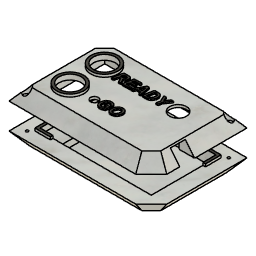
stopwatch_transmitter (Autodesk Fusion 360 design; units mm, degrees)
Autodesk Fusion 360 part; units mm, degrees
note: some values were not read from the file. Chosen so that the rebuilt part matches the saved one: which face or edge a step refers to; which sketch regions a step uses; which pieces of a blend or face edit are solid.
sketch "Sketch1" plane through (0, 0, 0) normal (0, 0, 1) x (1, 0, 0)
  line L0 (0, 0) -> (70, 0)
  line L1 (70, 0) -> (70, 50)
  line L2 (70, 50) -> (0, 50)
  line L3 (0, 50) -> (0, 0)
  line L4 (-2, -2) -> (72, -2)
  line L5 (72, -2) -> (72, 52)
  line L6 (72, 52) -> (-2, 52)
  line L7 (-2, 52) -> (-2, -2)
  line L8 (0, 50) -> (-14, 50)
  line L9 (-14, 50) -> (-14, 0)
  line L10 (-14, 0) -> (0, 0)
  line L11 (0, 0) -> (0, 50)
  line L12 (2, 52) -> (-16, 52)
  line L13 (-16, 52) -> (-16, -2)
  line L14 (-16, -2) -> (2, -2)
  dimension "d1" = 70
  dimension "d2" = 50
  dimension "d3" = 2
  dimension "d10" = 14
  constraint horizontal L0
  constraint vertical L1
  constraint horizontal L2
  constraint vertical L3
  constraint coincident L0.start L3.end
  constraint horizontal L8
  constraint vertical L9
  constraint horizontal L10
  constraint vertical L11
  measures "d1" distance of L0.start L0.end
  measures "d2" distance of L0.start L2.end
  measures "d10" distance of L2.end L8.end
extrude "Extrude1" add sketch "Sketch1" along normal blind 2 contours L0 L1 L2 L3 L11 makes body 1
extrude "Extrude2" add sketch "Sketch1" along normal blind 5 contours L3 L7 L8 L10 L11 | L0 L1 L2 L4 L5 L6 L7 L8 L10 L12 L14 bodies 1
extrude "Extrude3" add 1 faces at (46.6667, -1.3333, 5) along direction (0, 0, 1) blind 2 on bodies 1 bodies 1
extrude "Extrude4" add sketch "Sketch1" along normal blind 8 contours L7 L8 L9 L10 L12 L13 L14 bodies 1
extrude "Extrude5" add sketch "Sketch1" along normal blind 7 contours L7 L8 L9 L10 bodies 1
sketch "Sketch2" plane through (0, 0, 7) normal (0, 0, 1) x (-1, 0, 0)
  line L0 (0, 0) -> (0, -50)
  line L1 (0, -50) -> (-70, -50)
  line L2 (-70, -50) -> (-70, 0)
  line L3 (-70, 0) -> (0, 0)
  line L4 (2, -52) -> (2, -50)
  line L5 (2, -50) -> (14, -50)
  line L6 (14, -50) -> (14, 0)
  line L7 (14, 0) -> (2, 0)
  line L8 (2, 0) -> (2, 2)
  line L9 (2, 2) -> (-72, 2)
  line L10 (-72, 2) -> (-72, -52)
  line L11 (-72, -52) -> (2, -52)
  line L12 (0, 0) -> (2, 0)
  line L13 (0, -50) -> (2, -50)
  constraint coincident L0.start L3.end
  constraint coincident L7.end L8.start
  constraint coincident L0.end L1.start
  constraint coincident L4.end L5.start
extrude "Extrude6" add sketch "Sketch2" along normal blind 1 contours L1 L2 L3 L4 L8 L9 L10 L11 L12 L13 bodies 1
extrude "Extrude7" add 1 faces at (72, 16, 2.6667) along direction (1, 0, 0) blind 1 on bodies 1 bodies 1
sketch "Sketch3" plane through (0, 0, 8) normal (0, 0, 1) x (-1, 0, 0)
  line L0 (-73, -52) -> (16, -52)
  line L1 (16, -52) -> (16, 2)
  line L2 (16, 2) -> (-73, 2)
  line L3 (-73, 2) -> (-73, -52)
  line L4 (14, -50) -> (-70, -50)
  line L5 (-70, -50) -> (-70, 0)
  line L6 (-70, 0) -> (14, 0)
  line L7 (14, 0) -> (14, -50)
  line L8 (-70, -50) -> (-71, -50)
  line L9 (-71, -50) -> (-71, 0)
  line L10 (-71, 0) -> (-70, 0)
  line L11 (-70, 0) -> (-70, -50)
  line L12 (-70, -50) -> (-71, -50)
  line L13 (-71, -50) -> (-71, -30)
  line L14 (-71, -30) -> (-70, -30)
  line L15 (-70, -30) -> (-70, -50)
  line L16 (-71, 0) -> (-70, 0)
  line L17 (-70, 0) -> (-70, -20)
  line L18 (-70, -20) -> (-71, -20)
  line L19 (-71, -20) -> (-71, 0)
  dimension "d20" = 1
  dimension "d21" = 20
  constraint horizontal L8
  constraint vertical L9
  constraint horizontal L10
  constraint vertical L11
  constraint coincident L4.end L5.start
  constraint horizontal L12
  constraint vertical L13
  constraint horizontal L14
  constraint vertical L15
  constraint coincident L9 L13.end
  constraint horizontal L16
  constraint vertical L17
  constraint horizontal L18
  constraint vertical L19
  measures "d20" distance of L4.end L8.end
  measures "d21" distance of L9.end L18.end
extrude "Extrude8" cut sketch "Sketch3" against normal blind 1 contours L5 L8 L9 L11 L12 L13 L14 L15 | L5 L9 L10 L11 L16 L17 L18 L19 bodies 1
extrude "Extrude9" cut sketch "Sketch3" against normal blind 6 contours L5 L9 L11 L14 L18 bodies 1
extrude "Extrude10" add 1 faces at (73, 16, 2.6667) along direction (1, 0, 0) blind 1 on bodies 1 bodies 1
extrude "Extrude11" cut 1 faces at (71, 26.6667, 3.6667) along direction (1, 0, 0) blind 1 on bodies 1 bodies 1
sketch "Sketch4" plane through (0, 0, 8) normal (0, 0, 1) x (-1, 0, 0)
  line L0 (-72, 0) -> (14, 0)
  line L1 (14, 0) -> (14, -50)
  line L2 (14, -50) -> (-72, -50)
  line L3 (-72, -50) -> (-72, 0)
  line L4 (-74, -52) -> (16, -52)
  line L5 (16, -52) -> (16, 2)
  line L6 (16, 2) -> (-74, 2)
  line L7 (-74, 2) -> (-74, -52)
  line L8 (16, -52) -> (-74, -52)
  line L9 (-74, 2) -> (16, 2)
  line L10 (16, 2) -> (16, -52)
  line L11 (-74, 2) -> (-74, 1.5)
  line L12 (-74, 2) -> (-74, -10)
  line L13 (-74, -52) -> (-74, -21)
  line L14 (-74, -21) -> (-72, -21)
  line L15 (-72, -21) -> (-72, -10)
  line L16 (-72, -10) -> (-74, -10)
  line L17 (16, -52) -> (-10.5, -52)
  line L18 (-74, -52) -> (-19.5, -52)
  line L19 (-10.5, -52) -> (-19.5, -52)
  line L20 (-19.5, -52) -> (-19.5, -50)
  line L21 (-19.5, -50) -> (-10.5, -50)
  line L22 (-10.5, -50) -> (-10.5, -52)
  line L23 (16, -52) -> (16, -47)
  line L24 (16, 2) -> (16, -3)
  line L25 (16, -25) -> (16, -30)
  line L26 (16, -25) -> (16, -20)
  line L27 (16, 2) -> (15, 2)
  line L28 (16, 2) -> (11, 2)
  line L29 (16, -52) -> (11, -52)
  line L30 (-74, -52) -> (-73.5, -52)
  line L31 (-74, -52) -> (-63, -52)
  line L32 (-74, -52) -> (-74, -42)
  line L33 (16, 2) -> (-12, 2)
  line L34 (16, 2) -> (16, -9)
  line L35 (2.5, -38.5) -> (2.5, -38.25)
  circle A0 centre (2.5, -38.25) radius 8.5
  line L36 (2.5, -11.5) -> (2.5, -11.75)
  circle A1 centre (2.5, -11.75) radius 8.5
  line L37 (-15, -12) -> (-16, -12)
  line L38 (-56.5, -35.5) -> (-56.5, -36.5)
  line L39 (-56.5, -36.5) -> (-56.25, -36.5)
  circle A2 centre (-56.25, -36.5) radius 6.5
  circle A3 centre (-16, -12) radius 3
  line L40 (-8.9387, -32.2692) -> (-47.6004, -32.6117) construction
  line L41 (-47.6004, -32.6117) -> (-47.5301, -40.5565) construction
  line L42 (-47.5301, -40.5565) -> (-8.8683, -40.214) construction
  line L43 (-8.8683, -40.214) -> (-8.9387, -32.2692) construction
  line L44 (-20.8588, -8.0842) -> (-38.0381, -8.2489) construction
  line L45 (-38.0381, -8.2489) -> (-37.9619, -16.1956) construction
  line L46 (-37.9619, -16.1956) -> (-20.7826, -16.0308) construction
  line L47 (-20.7826, -16.0308) -> (-20.8588, -8.0842) construction
  circle A4 centre (2.5, -38.25) radius 10.5
  circle A5 centre (2.5, -11.75) radius 10.5
  dimension "d30" = 12
  dimension "d31" = 31
  dimension "d32" = 26.5
  dimension "d33" = 54.5
  dimension "d34" = 5
  dimension "d35" = 5
  dimension "d36" = 5
  dimension "d37" = 5
  dimension "d38" = 5
  dimension "d41" = 5
  dimension "d44" = 11
  dimension "d45" = 10
  dimension "d48" = 28
  dimension "d49" = 11
  dimension "d58" = 0.25
  dimension "d59" = 17
  dimension "d60" = 0.25
  dimension "d61" = 17
  dimension "d64" = 1
  dimension "d65" = 1
  dimension "d66" = 0.25
  dimension "d67" = 13
  dimension "d68" = 6
  dimension "d75" = 8
  dimension "d76" = 8
  dimension "d77" = 2
  dimension "d78" = 2
  text T0 "READY" font "Arial" height 8 bold italic align left top in box 38.6633 x 7.9451 at (-8.9387, -32.2692) x (-0.999961, -0.00886) y (0.00886, -0.999961) spacing 1
  text T1 "GO" font "Arial" height 8 bold italic align left top in box 17.1801 x 7.947 at (-20.8588, -8.0842) x (-0.999954, -0.00959) y (0.00959, -0.999954) spacing 1
  constraint horizontal L8
  constraint horizontal L9
  constraint vertical L10
  constraint coincident L6.end L7.start
  constraint coincident L4.end L5.start
  constraint perpendicular L9 L12
  constraint perpendicular L4 L13
  constraint horizontal L14
  constraint vertical L15
  constraint horizontal L16
  constraint coincident L3 L15.end
  constraint perpendicular L1 L17
  constraint perpendicular L13 L18
  constraint horizontal L19
  constraint vertical L20
  constraint horizontal L21
  constraint vertical L22
  constraint coincident L2 L20.end
  constraint perpendicular L17 L23
  constraint coincident L5.end L6.start
  constraint perpendicular L0 L24
  constraint midpoint L10 L25.start
  constraint parallel L10 L25
  constraint parallel L5 L26
  constraint coincident L9 L27.end
  constraint perpendicular L10 L27
  constraint perpendicular L10 L28
  constraint perpendicular L10 L29
  constraint coincident L18 L30.end
  constraint perpendicular L13 L30
  constraint coincident L4.start L7.end
  constraint perpendicular L7 L31
  constraint perpendicular L31 L32
  constraint perpendicular L24 L33
  constraint perpendicular L0 L34
  constraint vertical L35
  constraint coincident L35.end A0.centre
  constraint vertical L36
  constraint coincident L36.end A1.centre
  constraint horizontal L37
  constraint vertical L38
  constraint perpendicular L38 L39
  constraint coincident L39.end A2.centre
  constraint coincident L37.end A3.centre
  measures "d30" distance of L6.end L12.end
  measures "d31" distance of L4.start L13.end
  measures "d32" distance of L4.end L17.end
  measures "d33" distance of L4.start L18.end
  measures "d34" distance of L4.end L23.end
  measures "d35" distance of L5.end L24.end
  measures "d36" distance of L25.start L25.end
  measures "d37" distance of L25.start L26.end
  measures "d38" distance of L5.end L28.end
  measures "d41" distance of L4.end L29.end
  measures "d44" distance of L4.start L31.end
  measures "d45" distance of L4.start L32.end
  measures "d48" distance of L5.end L33.end
  measures "d49" distance of L5.end L34.end
  measures "d58" distance of L35.start L35.end
  measures "d59" diameter of A0
  measures "d60" distance of L36.start L36.end
  measures "d61" diameter of A1
  measures "d64" distance of L37.start L37.end
  measures "d65" distance of L38.start L38.end
  measures "d66" distance of L38.end L39.end
  measures "d67" diameter of A2
  measures "d68" diameter of A3
extrude "Extrude12" add sketch "Sketch4" along normal blind 2 separate body contours L0 L1 L2 L3 L4 L5 L6 L7 L8 L9 L10 L11 L12 L16 L17 L22 L23 L24 L25 L26 L27 L28 L29 L33 L34 | L0 L1 L2 L3 L15 L21 | L2 L3 L4 L7 L8 L13 L14 L18 L20 L30 L31 L32 | A0 | A1 | A2 | A3 | A4 | A5 makes body 2
extrude "Extrude13" cut 1 faces at (73.3333, 21, 8.6667) along direction (0, 1, 0) blind 0.5 on bodies 2 bodies 2
extrude "Extrude14" add sketch "Sketch4" along normal blind 2 contours A5 bodies 2
extrude "Extrude15" add sketch "Sketch4" along normal blind 2 contours A5 bodies 2
extrude "Extrude16" cut sketch "Sketch4" along normal blind 16 contours A0 | A1 | A2 | A3 bodies 2
extrude "Extrude17" add 1 faces at (0, 33.3333, 3.6667) along direction (1, 0, 0) blind 1 on bodies 1 bodies 1
extrude "Extrude18" add 1 faces at (14.6667, -1.3333, 8) along direction (0, 0, 1) blind 0.5 on bodies 1 bodies 1
extrude "Extrude19" add sketch "Sketch4" sketch "Sketch4" along normal blind 3 contours A4 | A5 of sketch 2 text T0 T1 bodies 2
extrude "Extrude20" add 2 faces at (-12.2942, 38.7716, 11) (-12.2626, 12.6939, 11) along direction (0, 0, 1) blind 1 on bodies 2 bodies 2
move_body "Move1" bodies 2 to x (1, 0, 0) y (0, 1, 0) z (0, 0, 1) at (0, 0, 9)
extrude "Extrude21" add sketch "Sketch4" along normal blind 9 separate body contours L0 L1 L2 L3 L4 L5 L6 L7 L8 L9 L10 L11 L12 L16 L17 L22 L23 L24 L25 L26 L27 L28 L29 L33 L34 | L2 L3 L4 L7 L8 L13 L14 L18 L20 L30 L31 L32 makes body 3 at (14, -2, 14) makes body 4 at (55.8333, 52, 11)
combine "Combine1" operation add target body 3 tool bodies 2 4
extrude "Extrude22" cut 1 faces at (73.3333, 21, 11) along direction (0, 1, 0) blind 0.5 on bodies 3 bodies 3
extrude "Extrude23" add 2 faces at (72, 17.3333, 18.3333) (72, 21.1667, 17.6667) along direction (1, 0, 0) blind 2 on bodies 3 bodies 3
extrude "Extrude24" add 1 faces at (13.5, 50, 17.6667) along direction (0, 1, 0) blind 2 on bodies 3 bodies 3
move_body "Move2" bodies 3 to x (1, 0, 0) y (0, 1, 0) z (0, 0, 1) at (0, 0, 5)
extrude "Extrude25" add 1 faces at (14.6667, -1.3333, 8.5) along direction (0, 0, 1) blind 1 on bodies 1 bodies 1
move_body "Move3" bodies 1 to x (1, 0, 0) y (0, 1, 0) z (0, 0, 1) at (0, 0, -3)
extrude "Extrude26" cut sketch "Sketch4" against normal blind 2.5 contours L3 L7 L14 L15 L16 bodies 1
extrude "Extrude27" cut 1 faces at (73.3333, 21, 6.1667) along direction (0, 1, 0) blind 0.5 on bodies 1 bodies 1
extrude "Extrude28" cut 2 faces at (43.3333, -1.3333, 13) (55.1667, 51.3333, 13) along direction (0, 0, 1) blind 1 on bodies 3 bodies 3
extrude "Extrude29" add 1 faces at (44, 16, -3) along direction (0, 0, -1) blind 0.5 on bodies 1 bodies 1
extrude "Extrude30" cut sketch "Sketch4" against normal blind 3 contours L2 L4 L8 L19 L20 L21 L22 bodies 1
sketch "Sketch5" plane through (0, 0, 22) normal (0, 0, -1) x (1, 0, 0)
  circle A0 centre (56.25, -36.5) radius 6.5
  circle A1 centre (16, -12) radius 3
  circle A2 centre (-2.5, -11.75) radius 8.5
  circle A3 centre (-2.5, -38.25) radius 8.5
  line L0 (19.5, -50) -> (72, -50)
  line L1 (72, -50) -> (72, -21.5)
  line L2 (72, -21.5) -> (74, -21.5)
  line L3 (74, -21.5) -> (74, -10)
  line L4 (74, -10) -> (72, -10)
  line L5 (72, -10) -> (72, 0)
  line L6 (72, 0) -> (-14, 0)
  line L7 (-14, 0) -> (-14, -50)
  line L8 (-14, -50) -> (10.5, -50)
  line L9 (10.5, -50) -> (10.5, -52)
  line L10 (10.5, -52) -> (19.5, -52)
  line L11 (19.5, -52) -> (19.5, -50)
  line L12 (19.5, -52) -> (10.5, -52)
  line L13 (10.5, -52) -> (10.5, -50)
  line L14 (10.5, -50) -> (19.5, -50)
  line L15 (19.5, -50) -> (19.5, -52)
  constraint horizontal L12
  constraint vertical L13
  constraint horizontal L14
  constraint vertical L15
  constraint coincident L8.end L9.start
  constraint coincident L10.end L11.start
extrude "Extrude31" add sketch "Sketch5" along normal blind 0.5 contours L9 L10 L11 L12 L13 L14 L15 bodies 3
move_body "Move4" bodies 3 to x (1, 0, 0) y (0, 1, 0) z (0, 0, 1) at (0, 0, -7.5)
extrude "Extrude32" add 1 faces at (13.5, 50.6667, 14) along direction (0, 0, -1) blind 2 on bodies 3 bodies 3
extrude "Extrude33" add 1 faces at (19.5, 51.3333, 8.3333) along direction (-1, 0, 0) blind 1 on bodies 3 bodies 3
extrude "Extrude34" add 1 faces at (10.5, 50.6667, 8.3333) along direction (1, 0, 0) blind 1 on bodies 3 bodies 3
extrude "Extrude35" add 1 faces at (19.5, 51.3333, 6) along direction (-1, 0, 0) blind 1 on bodies 1 bodies 1
extrude "Extrude36" add 1 faces at (10.5, 50.6667, 6) along direction (1, 0, 0) blind 1 on bodies 1 bodies 1
extrude "Extrude37" cut 1 faces at (11.5, 50.6667, 6) along direction (-1, 0, 0) blind 0.5 on bodies 1 bodies 1
extrude "Extrude38" add 1 faces at (11, 50.6667, 6) along direction (1, 0, 0) blind 0.25 on bodies 1 bodies 1
extrude "Extrude39" cut 1 faces at (11.5, 50.6667, 8.3333) along direction (-1, 0, 0) blind 0.25 on bodies 3 bodies 3
extrude "Extrude40" add 1 faces at (73.3333, 17.5, 5.5) along direction (0, 0, 1) blind 1 on bodies 1 bodies 1
extrude "Extrude41" add 1 faces at (14, -2, 9.8333) along direction (0, -1, 0) blind 10 on bodies 3 bodies 3
extrude "Extrude42" add 4 faces at (74, -4.6667, 12.5) (74, 13.6667, 15.8333) (74, 41.8333, 12.5) (74, 21.3333, 15.8333) along direction (1, 0, 0) blind 10 on bodies 3 bodies 3
extrude "Extrude43" add 1 faces at (62.1667, 52, 11.6667) along direction (0, 1, 0) blind 10 on bodies 3 bodies 3
extrude "Extrude44" add 1 faces at (-16, 37.3333, 13.1667) along direction (-1, 0, 0) blind 10 on bodies 3 bodies 3
chamfer "Chamfer1" distance 12 angle 45 2 edges at (84, -12, 11.5) (-26, 62, 11.5) on bodies 3
chamfer "Chamfer2" distance 8 distance2 10 6 edges at (23, -12, 16.5) (78, -6, 16.5) (84, 31, 16.5) (35, 62, 16.5) (-20, 56, 16.5) (-26, 19, 16.5) measured on face at (35.4296, 54.819, 16.5) measured on face at (80, -4, 13.1667) measured on face at (35.4296, 54.819, 16.5) measured on face at (35.4296, 54.819, 16.5) measured on face at (-22, 54, 9.8333) measured on face at (-26, 8.6667, 9.8333) on bodies 3
move_face "OffsetFaces1" offset 10 4 faces at (44, -2, -0.1667) (74, 34, 3.1667) (55.5, 52, 2.6667) (-16, 34, -0.1667) on bodies 1
chamfer "Chamfer3" distance 12 distance2 12 2 edges at (-26, 62, 1.5) (84, -12, 1.5) measured on face at (62.1667, 62, 2.6667) measured on face at (10.6667, -12, 3.1667) on bodies 1
chamfer "Chamfer4" distance 8 distance2 10 6 edges at (23, -12, -3.5) (78, -6, -3.5) (84, 31, -3.5) (35, 62, -3.5) (-20, 56, -3.5) (-26, 19, -3.5) measured on face at (47.3333, 37.3333, -3.5) measured on face at (80, -4, -0.1667) measured on face at (47.3333, 37.3333, -3.5) measured on face at (47.3333, 37.3333, -3.5) measured on face at (-18, 58, -0.1667) measured on face at (47.3333, 37.3333, -3.5) on bodies 1
move_body "Move5" bodies 3 to x (1, 0, 0) y (0, 1, 0) z (0, 0, 1) at (0, 0, 20)
sketch "Sketch6" plane through (0, 0, 6.5) normal (0, 0, 1) x (-1, 0, 0)
  line L0 (-72, 12) -> (-84, 0)
  line L1 (-84, 0) -> (-84, -62)
  line L2 (-84, -62) -> (-18.5, -62)
  line L3 (-18.5, -62) -> (-18.5, -50)
  line L4 (-18.5, -50) -> (-72, -50)
  line L5 (-72, -50) -> (-72, 0)
  line L6 (-72, 0) -> (14, 0)
  line L7 (14, 0) -> (14, -50)
  line L8 (14, -50) -> (-11.25, -50)
  line L9 (-11.25, -50) -> (-11.25, -62)
  line L10 (-11.25, -62) -> (14, -62)
  line L11 (14, -62) -> (26, -50)
  line L12 (26, -50) -> (26, 12)
  line L13 (26, 12) -> (-72, 12)
  line L14 (14, 0) -> (16, 0)
  line L15 (16, 0) -> (16, -10)
  line L16 (16, -10) -> (14, -10)
  line L17 (14, -10) -> (14, 0)
  line L18 (16, 0) -> (4, 0)
  line L19 (4, 0) -> (4, 2)
  line L20 (4, 2) -> (16, 2)
  line L21 (16, 2) -> (16, 0)
  line L22 (-72, -50) -> (-62, -50)
  line L23 (-62, -50) -> (-62, -52)
  line L24 (-62, -52) -> (-72, -52)
  line L25 (-72, -52) -> (-72, -50)
  line L26 (-72, -52) -> (-74, -52)
  line L27 (-74, -52) -> (-74, -40)
  line L28 (-74, -40) -> (-72, -40)
  line L29 (-72, -40) -> (-72, -52)
  dimension "d139" = 2
  dimension "d140" = 10
  dimension "d141" = 12
  dimension "d142" = 2
  dimension "d143" = 10
  dimension "d144" = 2
  dimension "d145" = 2
  dimension "d146" = 12
  constraint horizontal L14
  constraint vertical L15
  constraint horizontal L16
  constraint vertical L17
  constraint coincident L6.end L7.start
  constraint horizontal L18
  constraint vertical L19
  constraint horizontal L20
  constraint vertical L21
  constraint horizontal L22
  constraint vertical L23
  constraint horizontal L24
  constraint vertical L25
  constraint coincident L4.end L5.start
  constraint horizontal L26
  constraint vertical L27
  constraint horizontal L28
  constraint vertical L29
  measures "d139" distance of L6.end L14.end
  measures "d140" distance of L6.end L16.end
  measures "d141" distance of L14.end L18.end
  measures "d142" distance of L14.end L20.end
  measures "d143" distance of L4.end L22.end
  measures "d144" distance of L4.end L24.end
  measures "d145" distance of L24.end L26.end
  measures "d146" distance of L24.end L28.end
extrude "Extrude45" add sketch "Sketch6" along normal blind 2 contours L7 L14 L15 L16 L17 L18 | L6 L14 L18 L19 L20 L21 bodies 1
extrude "Extrude46" add sketch "Sketch6" along normal blind 2 contours L4 L22 L23 L24 L25 L29 | L5 L25 L26 L27 L28 L29 bodies 1
extrude "Extrude47" cut sketch "Sketch6" along normal blind 28 contours L4 L22 L23 L24 L25 L29 | L5 L25 L26 L27 L28 L29 | L7 L14 L15 L16 L17 L18 | L6 L14 L18 L19 L20 L21 bodies 3
extrude "Extrude48" cut 1 faces at (-15.3333, 10, 29.1667) along direction (0, 1, 0) blind 1 on bodies 3 bodies 3
extrude "Extrude49" cut 1 faces at (-4, -0.6667, 29.1667) along direction (1, 0, 0) blind 1 on bodies 3 bodies 3
extrude "Extrude50" cut 1 faces at (62, 50.6667, 29.1667) along direction (-1, 0, 0) blind 1 on bodies 3 bodies 3
extrude "Extrude51" cut 1 faces at (73.3333, 40, 29.1667) along direction (0, -1, 0) blind 1 on bodies 3 bodies 3
sketch "Sketch7" plane through (0, 0, 6.5) normal (0, 0, 1) x (-1, 0, 0)
  line L0 (-62, -50) -> (-62, -52)
  line L1 (-62, -52) -> (-74, -52)
  line L2 (-74, -52) -> (-74, -40)
  line L3 (-74, -40) -> (-72, -40)
  line L4 (-72, -40) -> (-72, 0)
  line L5 (-72, 0) -> (4, 0)
  line L6 (4, 0) -> (4, 2)
  line L7 (4, 2) -> (16, 2)
  line L8 (16, 2) -> (16, -10)
  line L9 (16, -10) -> (14, -10)
  line L10 (14, -10) -> (14, -50)
  line L11 (14, -50) -> (-11.25, -50)
  line L12 (-11.25, -50) -> (-11.25, -62)
  line L13 (-11.25, -62) -> (14, -62)
  line L14 (14, -62) -> (26, -50)
  line L15 (26, -50) -> (26, 12)
  line L16 (26, 12) -> (-72, 12)
  line L17 (-72, 12) -> (-84, 0)
  line L18 (-84, 0) -> (-84, -62)
  line L19 (-84, -62) -> (-18.5, -62)
  line L20 (-18.5, -62) -> (-18.5, -50)
  line L21 (-18.5, -50) -> (-62, -50)
  line L22 (16, 2) -> (22, 2)
  line L23 (22, 2) -> (22, 8)
  line L24 (22, 8) -> (16, 8)
  line L25 (16, 8) -> (16, 2)
  circle A0 centre (19, 5) radius 1
  circle A1 centre (19, 5) radius 3
  line L26 (-74, -52) -> (-80, -52)
  line L27 (-80, -52) -> (-80, -58)
  line L28 (-80, -58) -> (-74, -58)
  line L29 (-74, -58) -> (-74, -52)
  circle A2 centre (-77, -55) radius 1
  circle A3 centre (-77, -55) radius 3
  dimension "d161" = 6
  dimension "d162" = 6
  dimension "d163" = 2
  dimension "d164" = 6
  dimension "d165" = 6
  dimension "d166" = 2
  constraint horizontal L22
  constraint vertical L23
  constraint horizontal L24
  constraint vertical L25
  constraint coincident L7.end L8.start
  constraint concentric A0 A1
  constraint tangent L25 A1
  constraint horizontal L26
  constraint vertical L27
  constraint horizontal L28
  constraint vertical L29
  constraint coincident L1.end L2.start
  constraint concentric A2 A3
  constraint tangent L27 A3
  measures "d161" distance of L7.end L22.end
  measures "d162" distance of L7.end L24.end
  measures "d163" diameter of A0
  measures "d164" distance of L1.end L26.end
  measures "d165" distance of L1.end L28.end
  measures "d166" diameter of A2
extrude "Extrude52" cut sketch "Sketch7" against normal blind 4 contours A0 bodies 1
extrude "Extrude53" cut sketch "Sketch7" against normal blind 4 contours A2 bodies 1
extrude "Extrude54" cut sketch "Sketch7" along normal blind 57 contours A0 | A2 bodies 3
sketch "Sketch8" plane through (0, 0, 36.5) normal (0, 0, 1) x (-1, 0, 0)
  line L0 (-10.5871, -32.2289) -> (-8.9392, -32.2143)
  line L1 (-8.9392, -32.2143) -> (-10.5435, -40.2288)
  line L2 (-10.5435, -40.2288) -> (-14.0959, -40.2603)
  spline S0 degree 3 poles (-14.0959, -40.2603) (-14.3379, -40.2599) (-14.5799, -40.2596) (-15.0631, -40.2046) (-15.2587, -40.1538) (-15.5245, -40.0847) knots 0 0 0 0 0.072595 0.072595 0.147152 0.147152 0.147152 0.147152
  spline S1 degree 3 poles (-15.5245, -40.0847) (-15.699, -40.0034) (-15.8595, -39.9287) (-16.1355, -39.6999) (-16.245, -39.5508) (-16.3546, -39.4017) knots 0 0 0 0 0.05773 0.05773 0.115402 0.115402 0.115402 0.115402
  spline S2 degree 3 poles (-16.3546, -39.4017) (-16.4602, -39.1966) (-16.5501, -39.022) (-16.6558, -38.6156) (-16.6675, -38.4016) (-16.6792, -38.1876) knots 0 0 0 0 0.069205 0.069205 0.138098 0.138098 0.138098 0.138098
  spline S3 degree 3 poles (-16.6792, -38.1876) (-16.6609, -37.8769) (-16.6425, -37.5662) (-16.4471, -37.0013) (-16.2758, -36.7649) (-16.0829, -36.4987) knots 0 0 0 0 0.093372 0.093372 0.18695 0.18695 0.18695 0.18695
  spline S4 degree 3 poles (-16.0829, -36.4987) (-15.7851, -36.2497) (-15.5518, -36.0546) (-14.9295, -35.7821) (-14.5849, -35.7216) (-14.2403, -35.6611) knots 0 0 0 0 0.116479 0.116479 0.231434 0.231434 0.231434 0.231434
  spline S5 degree 3 poles (-14.2403, -35.6611) (-14.365, -35.5388) (-14.4682, -35.4374) (-14.6683, -35.1883) (-14.755, -35.0536) (-14.8418, -34.9188) knots 0 0 0 0 0.052389 0.052389 0.104433 0.104433 0.104433 0.104433
  spline S6 degree 3 poles (-14.8418, -34.9188) (-15.1074, -34.4325) (-15.3033, -34.074) (-15.7224, -33.1803) (-15.9077, -32.729) (-16.093, -32.2777) knots 0 0 0 0 0.166241 0.166241 0.328188 0.328188 0.328188 0.328188
  line L3 (-16.093, -32.2777) -> (-14.325, -32.262)
  spline S7 degree 3 poles (-14.325, -32.262) (-14.177, -32.6697) (-14.0732, -32.9555) (-13.7789, -33.6741) (-13.6252, -34.0202) (-13.4714, -34.3664) knots 0 0 0 0 0.130111 0.130111 0.253846 0.253846 0.253846 0.253846
  spline S8 degree 3 poles (-13.4714, -34.3664) (-13.3816, -34.5624) (-13.2918, -34.7583) (-13.0498, -35.1139) (-12.921, -35.2345) (-12.7419, -35.4023) knots 0 0 0 0 0.064675 0.064675 0.131653 0.131653 0.131653 0.131653
  spline S9 degree 3 poles (-12.7419, -35.4023) (-12.5926, -35.4652) (-12.4876, -35.5095) (-12.2064, -35.5556) (-12.0642, -35.5544) (-11.922, -35.5532) knots 0 0 0 0 0.048618 0.048618 0.094938 0.094938 0.094938 0.094938
  line L4 (-11.922, -35.5532) -> (-11.2508, -35.5473)
  line L5 (-11.2508, -35.5473) -> (-10.5871, -32.2289)
  line L6 (-44.594, -32.5302) -> (-42.9515, -32.5156)
  line L7 (-42.9515, -32.5156) -> (-43.5732, -35.6372)
  line L8 (-43.5732, -35.6372) -> (-41.3254, -40.5016)
  line L9 (-41.3254, -40.5016) -> (-43.077, -40.5171)
  line L10 (-43.077, -40.5171) -> (-44.0902, -38.2668)
  spline S10 degree 3 poles (-44.0902, -38.2668) (-44.1764, -38.0741) (-44.2626, -37.8815) (-44.4301, -37.4811) (-44.4898, -37.3236) (-44.5753, -37.0977) knots 0 0 0 0 0.063314 0.063314 0.130264 0.130264 0.130264 0.130264
  spline S11 degree 3 poles (-44.5753, -37.0977) (-44.6538, -37.2346) (-44.7223, -37.354) (-44.8769, -37.6067) (-44.9574, -37.7308) (-45.0379, -37.8549) knots 0 0 0 0 0.047317 0.047317 0.094492 0.094492 0.094492 0.094492
  line L11 (-45.0379, -37.8549) -> (-45.7871, -38.9203)
  line L12 (-45.7871, -38.9203) -> (-46.9023, -40.551)
  line L13 (-46.9023, -40.551) -> (-48.8121, -40.5679)
  line L14 (-48.8121, -40.5679) -> (-45.1898, -35.4988)
  line L15 (-45.1898, -35.4988) -> (-44.594, -32.5302)
  line L16 (-29.6539, -34.166) -> (-26.4835, -34.1379)
  line L17 (-26.4835, -34.1379) -> (-25.5388, -32.3614)
  line L18 (-25.5388, -32.3614) -> (-23.8472, -32.3464)
  line L19 (-23.8472, -32.3464) -> (-28.3, -40.3861)
  line L20 (-28.3, -40.3861) -> (-30.128, -40.4023)
  line L21 (-30.128, -40.4023) -> (-31.4976, -32.4142)
  line L22 (-31.4976, -32.4142) -> (-29.937, -32.4003)
  line L23 (-29.937, -32.4003) -> (-29.6539, -34.166)
  line L24 (-16.977, -32.2855) -> (-18.5759, -40.3)
  line L25 (-18.5759, -40.3) -> (-24.5075, -40.3525)
  line L26 (-24.5075, -40.3525) -> (-24.241, -39.0131)
  line L27 (-24.241, -39.0131) -> (-19.9574, -38.9752)
  line L28 (-19.9574, -38.9752) -> (-19.5916, -37.1547)
  line L29 (-19.5916, -37.1547) -> (-23.7333, -37.1914)
  line L30 (-23.7333, -37.1914) -> (-23.4668, -35.852)
  line L31 (-23.4668, -35.852) -> (-19.3251, -35.8153)
  line L32 (-19.3251, -35.8153) -> (-18.8423, -33.639)
  line L33 (-18.8423, -33.639) -> (-23.497, -33.6803)
  line L34 (-23.497, -33.6803) -> (-23.2251, -32.3409)
  line L35 (-23.2251, -32.3409) -> (-16.977, -32.2855)
  circle A0 centre (-56.25, -36.5) radius 6.5
  circle A1 centre (-16, -12) radius 3
  spline S12 degree 3 poles (-29.5109, -11.2521) (-29.5194, -11.5197) (-29.5269, -11.7571) (-29.5942, -12.2566) (-29.6518, -12.503) (-29.7094, -12.7493) knots 0 0 0 0 0.080324 0.080324 0.160466 0.160466 0.160466 0.160466
  spline S13 degree 3 poles (-29.7094, -12.7493) (-29.8049, -13.075) (-29.9004, -13.4006) (-30.1759, -14.014) (-30.3481, -14.2839) (-30.5404, -14.5855) knots 0 0 0 0 0.101809 0.101809 0.203811 0.203811 0.203811 0.203811
  spline S14 degree 3 poles (-30.5404, -14.5855) (-30.7436, -14.8355) (-30.9435, -15.0815) (-31.4191, -15.4942) (-31.6928, -15.6593) (-31.9665, -15.8243) knots 0 0 0 0 0.096655 0.096655 0.193306 0.193306 0.193306 0.193306
  spline S15 degree 3 poles (-31.9665, -15.8243) (-32.2978, -15.9707) (-32.5936, -16.1014) (-33.2519, -16.2555) (-33.5947, -16.2744) (-33.9376, -16.2934) knots 0 0 0 0 0.10865 0.10865 0.217084 0.217084 0.217084 0.217084
  spline S16 degree 3 poles (-33.9376, -16.2934) (-34.3858, -16.2666) (-34.834, -16.2397) (-35.6397, -15.9455) (-35.9697, -15.6874) (-36.3447, -15.3942) knots 0 0 0 0 0.134711 0.134711 0.269775 0.269775 0.269775 0.269775
  spline S17 degree 3 poles (-36.3447, -15.3942) (-36.6471, -15.0126) (-36.9082, -14.6832) (-37.2144, -13.8671) (-37.2482, -13.4127) (-37.2821, -12.9584) knots 0 0 0 0 0.146075 0.146075 0.29162 0.29162 0.29162 0.29162
  spline S18 degree 3 poles (-37.2821, -12.9584) (-37.2595, -12.5226) (-37.2378, -12.1061) (-37.0462, -11.2877) (-36.8785, -10.8951) (-36.7108, -10.5026) knots 0 0 0 0 0.130896 0.130896 0.261757 0.261757 0.261757 0.261757
  spline S19 degree 3 poles (-36.7108, -10.5026) (-36.508, -10.1406) (-36.3053, -9.7787) (-35.7744, -9.1638) (-35.4588, -8.9255) (-35.1131, -8.6645) knots 0 0 0 0 0.124462 0.124462 0.249077 0.249077 0.249077 0.249077
  spline S20 degree 3 poles (-35.1131, -8.6645) (-34.7417, -8.4651) (-34.394, -8.2785) (-33.6259, -8.0602) (-33.2184, -8.032) (-32.811, -8.0039) knots 0 0 0 0 0.126467 0.126467 0.252855 0.252855 0.252855 0.252855
  spline S21 degree 3 poles (-32.811, -8.0039) (-32.4787, -8.0161) (-32.1464, -8.0282) (-31.5161, -8.1871) (-31.2477, -8.3271) (-30.929, -8.4934) knots 0 0 0 0 0.099765 0.099765 0.200057 0.200057 0.200057 0.200057
  spline S22 degree 3 poles (-30.929, -8.4934) (-30.7015, -8.6613) (-30.4741, -8.8293) (-30.1096, -9.2439) (-29.9829, -9.4792) (-29.842, -9.7409) knots 0 0 0 0 0.084824 0.084824 0.169794 0.169794 0.169794 0.169794
  spline S23 degree 3 poles (-29.842, -9.7409) (-29.7488, -9.9845) (-29.6557, -10.2281) (-29.5445, -10.7318) (-29.5282, -10.984) (-29.5109, -11.2521) knots 0 0 0 0 0.078246 0.078246 0.156532 0.156532 0.156532 0.156532
  circle A2 centre (2.5, -11.75) radius 10.5
  circle A3 centre (2.5, -38.25) radius 10.5
  line L36 (-32.529, -32.4233) -> (-34.1333, -40.4378)
  line L37 (-34.1333, -40.4378) -> (-36.2888, -40.4569)
  spline S24 degree 3 poles (-36.2888, -40.4569) (-36.4808, -40.4593) (-36.6728, -40.4617) (-37.0762, -40.4573) (-37.2251, -40.4501) (-37.4404, -40.4398) knots 0 0 0 0 0.057618 0.057618 0.121077 0.121077 0.121077 0.121077
  spline S25 degree 3 poles (-37.4404, -40.4398) (-37.5918, -40.4225) (-37.7432, -40.4052) (-38.0401, -40.3413) (-38.174, -40.297) (-38.3289, -40.2458) knots 0 0 0 0 0.045721 0.045721 0.091606 0.091606 0.091606 0.091606
  spline S26 degree 3 poles (-38.3289, -40.2458) (-38.4572, -40.1905) (-38.5847, -40.1356) (-38.8224, -39.9949) (-38.9322, -39.9093) (-39.0421, -39.8237) knots 0 0 0 0 0.041911 0.041911 0.083822 0.083822 0.083822 0.083822
  spline S27 degree 3 poles (-39.0421, -39.8237) (-39.1516, -39.7222) (-39.2543, -39.627) (-39.4397, -39.4073) (-39.5194, -39.2864) (-39.5991, -39.1656) knots 0 0 0 0 0.044805 0.044805 0.089584 0.089584 0.089584 0.089584
  spline S28 degree 3 poles (-39.5991, -39.1656) (-39.6813, -39.0158) (-39.754, -38.8834) (-39.8752, -38.5864) (-39.9198, -38.4315) (-39.9644, -38.2766) knots 0 0 0 0 0.051251 0.051251 0.102379 0.102379 0.102379 0.102379
  spline S29 degree 3 poles (-39.9644, -38.2766) (-40.0064, -38.0837) (-40.0435, -37.9133) (-40.0879, -37.5448) (-40.0938, -37.3587) (-40.0997, -37.1727) knots 0 0 0 0 0.059209 0.059209 0.118274 0.118274 0.118274 0.118274
  spline S30 degree 3 poles (-40.0997, -37.1727) (-40.0866, -36.7757) (-40.0735, -36.3786) (-39.9187, -35.6106) (-39.7819, -35.266) (-39.6262, -34.8737) knots 0 0 0 0 0.119171 0.119171 0.238665 0.238665 0.238665 0.238665
  spline S31 degree 3 poles (-39.6262, -34.8737) (-39.466, -34.5725) (-39.3057, -34.2713) (-38.8983, -33.7348) (-38.6658, -33.5194) (-38.3989, -33.2721) knots 0 0 0 0 0.102358 0.102358 0.205039 0.205039 0.205039 0.205039
  spline S32 degree 3 poles (-38.3989, -33.2721) (-38.1526, -33.1017) (-37.9488, -32.9607) (-37.4548, -32.7331) (-37.1904, -32.6577) (-36.9261, -32.5823) knots 0 0 0 0 0.089856 0.089856 0.179108 0.179108 0.179108 0.179108
  spline S33 degree 3 poles (-36.9261, -32.5823) (-36.6277, -32.5317) (-36.4162, -32.4958) (-35.8791, -32.4539) (-35.6146, -32.4511) (-35.3501, -32.4483) knots 0 0 0 0 0.090785 0.090785 0.177801 0.177801 0.177801 0.177801
  line L38 (-35.3501, -32.4483) -> (-32.529, -32.4233)
  line L39 (-24.7418, -12.3415) -> (-28.3214, -12.3758)
  line L40 (-28.3214, -12.3758) -> (-27.634, -8.9366)
  spline S34 degree 3 poles (-27.634, -8.9366) (-27.3666, -8.7786) (-27.1453, -8.6478) (-26.6274, -8.413) (-26.3578, -8.3209) (-26.0882, -8.2287) knots 0 0 0 0 0.093199 0.093199 0.185772 0.185772 0.185772 0.185772
  spline S35 degree 3 poles (-26.0882, -8.2287) (-25.7819, -8.1431) (-25.4757, -8.0576) (-24.8518, -7.9569) (-24.5354, -7.942) (-24.2165, -7.927) knots 0 0 0 0 0.095397 0.095397 0.190795 0.190795 0.190795 0.190795
  spline S36 degree 3 poles (-24.2165, -7.927) (-23.8064, -7.937) (-23.3963, -7.9471) (-22.6262, -8.1538) (-22.325, -8.3378) (-21.9346, -8.5763) knots 0 0 0 0 0.123066 0.123066 0.248073 0.248073 0.248073 0.248073
  spline S37 degree 3 poles (-21.9346, -8.5763) (-21.5666, -8.9838) (-21.2603, -9.3228) (-20.9015, -10.2127) (-20.8651, -10.7181) (-20.8287, -11.2234) knots 0 0 0 0 0.164713 0.164713 0.328405 0.328405 0.328405 0.328405
  spline S38 degree 3 poles (-20.8287, -11.2234) (-20.8443, -11.6085) (-20.8599, -11.9936) (-21.0073, -12.7408) (-21.1391, -13.1027) (-21.2711, -13.4651) knots 0 0 0 0 0.115623 0.115623 0.231247 0.231247 0.231247 0.231247
  spline S39 degree 3 poles (-21.2711, -13.4651) (-21.4608, -13.8561) (-21.6505, -14.247) (-22.1692, -14.9206) (-22.4837, -15.1839) (-22.8344, -15.4775) knots 0 0 0 0 0.13036 0.13036 0.260959 0.260959 0.260959 0.260959
  spline S40 degree 3 poles (-22.8344, -15.4775) (-23.2243, -15.7046) (-23.5771, -15.9101) (-24.3805, -16.151) (-24.81, -16.1805) (-25.2395, -16.21) knots 0 0 0 0 0.135358 0.135358 0.270512 0.270512 0.270512 0.270512
  spline S41 degree 3 poles (-25.2395, -16.21) (-25.6376, -16.197) (-26.0358, -16.184) (-26.7849, -15.9836) (-27.0905, -15.8067) (-27.4693, -15.5874) knots 0 0 0 0 0.119516 0.119516 0.240144 0.240144 0.240144 0.240144
  spline S42 degree 3 poles (-27.4693, -15.5874) (-27.7635, -15.3091) (-28.0147, -15.0715) (-28.3866, -14.4448) (-28.4921, -14.0829) (-28.5977, -13.7209) knots 0 0 0 0 0.121507 0.121507 0.24249 0.24249 0.24249 0.24249
  line L41 (-28.5977, -13.7209) -> (-27.0661, -13.5316)
  spline S43 degree 3 poles (-27.0661, -13.5316) (-26.9955, -13.7271) (-26.9249, -13.9227) (-26.7066, -14.2637) (-26.5692, -14.3918) (-26.4042, -14.5458) knots 0 0 0 0 0.062357 0.062357 0.125103 0.125103 0.125103 0.125103
  spline S44 degree 3 poles (-26.4042, -14.5458) (-26.2159, -14.6577) (-26.0557, -14.753) (-25.6754, -14.8612) (-25.472, -14.87) (-25.2686, -14.8787) knots 0 0 0 0 0.065724 0.065724 0.131149 0.131149 0.131149 0.131149
  spline S45 degree 3 poles (-25.2686, -14.8787) (-25.0102, -14.8593) (-24.7518, -14.8399) (-24.2656, -14.6973) (-24.0397, -14.5746) (-23.8102, -14.45) knots 0 0 0 0 0.077741 0.077741 0.155485 0.155485 0.155485 0.155485
  spline S46 degree 3 poles (-23.8102, -14.45) (-23.5707, -14.2619) (-23.3668, -14.1018) (-23.0258, -13.6675) (-22.903, -13.4126) (-22.7802, -13.1576) knots 0 0 0 0 0.091363 0.091363 0.182313 0.182313 0.182313 0.182313
  spline S47 degree 3 poles (-22.7802, -13.1576) (-22.6669, -12.8393) (-22.5619, -12.5444) (-22.4437, -11.9115) (-22.4328, -11.586) (-22.4219, -11.2605) knots 0 0 0 0 0.101366 0.101366 0.202646 0.202646 0.202646 0.202646
  spline S48 degree 3 poles (-22.4219, -11.2605) (-22.4323, -10.9891) (-22.4427, -10.7178) (-22.5927, -10.2133) (-22.7222, -10.0241) (-22.8945, -9.7725) knots 0 0 0 0 0.081474 0.081474 0.164671 0.164671 0.164671 0.164671
  spline S49 degree 3 poles (-22.8945, -9.7725) (-23.1136, -9.6054) (-23.288, -9.4724) (-23.7419, -9.3215) (-23.9917, -9.312) (-24.2415, -9.3024) knots 0 0 0 0 0.082652 0.082652 0.164411 0.164411 0.164411 0.164411
  spline S50 degree 3 poles (-24.2415, -9.3024) (-24.4321, -9.3115) (-24.6082, -9.3198) (-24.9697, -9.3738) (-25.1479, -9.4184) (-25.326, -9.4629) knots 0 0 0 0 0.057216 0.057216 0.114381 0.114381 0.114381 0.114381
  spline S51 degree 3 poles (-25.326, -9.4629) (-25.4902, -9.5117) (-25.6545, -9.5606) (-25.9748, -9.6823) (-26.1146, -9.7491) (-26.283, -9.8295) knots 0 0 0 0 0.051404 0.051404 0.103137 0.103137 0.103137 0.103137
  line L42 (-26.283, -9.8295) -> (-26.5171, -11.0215)
  line L43 (-26.5171, -11.0215) -> (-24.4763, -11.0019)
  line L44 (-24.4763, -11.0019) -> (-24.7418, -12.3415)
  line L45 (-76, -3.3137) -> (-76, -54)
  line L46 (-76, -54) -> (10.6863, -54)
  line L47 (10.6863, -54) -> (18, -46.6863)
  line L48 (18, -46.6863) -> (18, 4)
  line L49 (18, 4) -> (-68.6863, 4)
  line L50 (-68.6863, 4) -> (-76, -3.3137)
  circle A4 centre (19, 5) radius 3
  circle A5 centre (-77, -55) radius 3
  dimension "d173" = 6
  dimension "d174" = 6
  measures "d173" diameter of A4
  measures "d174" diameter of A5
extrude "Extrude55" cut sketch "Sketch8" against normal blind 7 contours L45 L46 A5 | L45 L46 A5 | L48 L49 A4 | L48 L49 A4 bodies 3
sketch "Sketch9" plane through (0, 0, 34.5) normal (0, 0, -1) x (1, 0, 0)
  circle A0 centre (-2.5, -38.25) radius 8.5
  circle A1 centre (-2.5, -11.75) radius 8.5
  circle A2 centre (16, -12) radius 3
  circle A3 centre (56.25, -36.5) radius 6.5
  line L0 (77.6, -21.5) -> (77.6, -10)
  line L1 (77.6, -10) -> (72, -10)
  line L2 (72, -10) -> (72, 0)
  line L3 (72, 0) -> (-3, 0)
  line L4 (-3, 0) -> (-3, 2)
  line L5 (-3, 2) -> (-16, 2)
  line L6 (-16, 2) -> (-16, -11)
  line L7 (-16, -11) -> (-14, -11)
  line L8 (-14, -11) -> (-14, -50)
  line L9 (-14, -50) -> (61, -50)
  line L10 (61, -50) -> (61, -52)
  line L11 (61, -52) -> (74, -52)
  line L12 (74, -52) -> (74, -39)
  line L13 (74, -39) -> (72, -39)
  line L14 (72, -39) -> (72, -21.5)
  line L15 (72, -21.5) -> (77.6, -21.5)
  line L16 (77.6, -21.5) -> (72, -21.5)
  line L17 (72, -21.5) -> (72, -10)
  line L18 (72, -10) -> (77.6, -10)
  line L19 (77.6, -10) -> (77.6, -21.5)
  constraint horizontal L16
  constraint vertical L17
  constraint horizontal L18
  constraint vertical L19
  constraint coincident L1.end L2.start
  constraint coincident L0.start L15.end
extrude "Extrude56" cut sketch "Sketch9" against normal blind 1 contours L0 L1 L15 L16 L17 L18 L19 bodies 3
chamfer "Chamfer5" distance 1 angle 45 1 edges at (72, 15.75, 34.5) on bodies 3
named bodies: "BASE_trans_V2", "TOP", "TOP_trans_V3"
